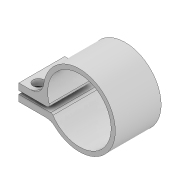
# Autodesk Inventor part: Halterung_Pumpe_210403
Saved by Autodesk Inventor 2020 (Build 240168000, 168)
## iProperties
Created: 2020-11-08
Part Number: Halterung_Pumpe_210403
Material: Generisch
Document SubType Name: Modeling
Designer: uhlma
Density: 1 g/cm^3
Appearance: Vorgabe
Author: uhlma
Autodesk Inventor part; units mm, degrees
ref_plane "YZ Plane" through (0, 0, 0) normal (1, 0, 0) x (0, 1, 0)
ref_plane "XZ Plane" through (0, 0, 0) normal (0, 1, 0) x (-1, 0, 0)
ref_plane "XY Plane" through (0, 0, 0) normal (0, 0, 1) x (1, 0, 0)
sketch "Skizze1" plane through (0, 0, 0) normal (0, 0, 1) x (1, 0, 0)
  arc A0 (-8.312, -5) -> (-8.8369, -4) centre (0, 0) ccw
  line L0 (-18.5, -7) -> (-8.4853, -7)
  line L1 (-18.5, -7) -> (-18.5, -5)
  line L2 (-18.5, -5) -> (-8.312, -5)
  line L3 (-18.5, -2) -> (-18.5, -4)
  line L4 (-18.5, -4) -> (-8.8369, -4)
  line L5 (-18.5, -2) -> (-14.8661, -2)
  arc A1 (-8.4853, -7) -> (-10.9018, 1.4667) centre (0, 0) ccw
  arc A2 (-14.8661, -2) -> (-10.9018, 1.4667) centre (-14.8661, 2) ccw
  point P0 (-10.8167, -2)
  dimension "d0" = 19.4
  dimension "d2" = 2
  dimension "d4" = 1
  dimension "d5" = 18.5
  dimension "d6" = 4
  dimension "d7" = 1.3
  dimension "d19" = 10.0147
  dimension "d27" = 4
  dimension "d28" = 3.6339
  constraints: 12 end point, 7 point on circle, 3 centre point, 3 point on line, 2 coincident, 2 perpendicular, 2 tangent, 1 collinear, 1 horizontal, 1 parallel, 1 vertical
  measures "d0" diameter of A0
  measures "d2" distance of L0.start L1.end
  measures "d4" distance between parallel lines of L4 L2
  measures "d5" distance from line of A1.centre L1
  measures "d6" distance edge to line of A1 L0
  measures "d7" radial gap between concentric circles of A1 A0
  measures "d19" distance of L0.end L0.start
  measures "d27" radius of A2
  measures "d28" distance of L3.start L5.end
extrude "Extrusion1" add sketch "Skizze1" along normal mid plane 14
sketch "Skizze2" plane through (-18.5, -2, 7) normal (0, 1, 0) x (1, 0, 0)
  circle A0 centre (3, 11) radius 1.65
  line L0 (0, 14) -> (3.6339, 14) projected
  line L1 (0, 14) -> (0, 0) projected
  line L2 (0, 14) -> (0, 0) construction
  line L3 (0, 7) -> (7.2294, 7) construction
  circle A1 centre (3, 3) radius 1.65
  circle A2 centre (3, 11) radius 3
  circle A3 centre (3, 3) radius 3
  point P0 (18.5, 7)
  point P1 (9.7894, 16)
  point P2 (0, 3)
  point P3 (0, 1.3417)
  point P4 (1.1676, 16)
  point P5 (0, 11)
  point P6 (0, 11.3417)
  point P7 (3, 14)
  dimension "d10" = 3
  dimension "d12" = 3.3
  dimension "d20" = 6
  dimension "d29" = 3
  constraints: 4 centre point, 2 coincident, 2 end point, 1 equal radius, 1 horizontal, 1 midpoint, 1 symmetric about line, 2 other
  measures "d12" diameter of A0
  measures "d20" diameter of A2
  measures "d29" distance from line of L1 A0.centre
extrude "Extrusion2" cut sketch "Skizze2" against normal through all both and the other way through all contours A0 | A1
fillet "Rundung2" radius 4 1 edges at (-8.4853, -7, 0)
fillet "Rundung3" radius 0.8 2 edges at (-8.8369, -4, 0) (-8.312, -5, 0)
extrude "Extrusion4" cut sketch "Skizze2" along normal blind 10 contours A3 | A2
